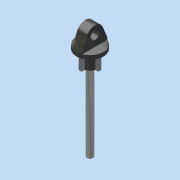
# Autodesk Inventor part: Shock Mount - Top
Saved by Autodesk Inventor 2011 SP1 (Build 150282100, 282)
## iProperties
Created: 2011-09-22
Part Number: Shock Mount - Top
Document SubType Name: Modeling
Designer: dgitz
Density: 1 g/cm^3
Author: dgitz
Autodesk Inventor part; units mm, degrees
ref_plane "YZ Plane" through (0, 0, 0) normal (1, 0, 0) x (0, 1, 0)
ref_plane "XZ Plane" through (0, 0, 0) normal (0, 1, 0) x (-1, 0, 0)
sketch "Sketch2" plane through (0, 0, 0) normal (0, 1, 0) x (-1, 0, 0)
  circle A0 centre (0, 0) radius 1.9812
  dimension "d0" = 3.9624
  constraints: 1 centre point, 1 coincident
  measures "d0" diameter of A0
extrude "Extrusion1" add sketch "Sketch2" along normal blind 50.8
chamfer "Chamfer1" distance 0.7937 angle 45 1 edges at (1.9812, 0, 0)
sketch "Sketch3" plane through (0, 50.8, 0) normal (0, 1, 0) x (1, 0, 0)
  circle A0 centre (0, 0) radius 1.9812 projected
  circle A1 centre (0, 0) radius 4.445
  dimension "d6" = 8.89
  constraints: 1 centre point, 1 coincident
  measures "d6" diameter of A1
extrude "Extrusion2" add sketch "Sketch3" along normal blind 8.89 contours A0 | A1
sketch "Sketch4" plane through (0, 59.69, 0) normal (0, 1, 0) x (1, 0, 0)
  circle A0 centre (0, 0) radius 4.445 projected
  circle A1 centre (0, 0) radius 8.509
  dimension "d9" = 17.018
  constraints: 1 centre point, 1 coincident
  measures "d9" diameter of A1
extrude "Extrusion3" add sketch "Sketch4" along normal blind 2.54 contours A0 | A1
sketch "Sketch5" plane through (0, 0, 0) normal (1, 0, 0) x (0, 1, 0)
  circle A0 centre (68.707, 0) radius 2.667
  arc A1 (70.7539, -5.0629) -> (70.7539, 5.0629) centre (68.707, 0) ccw
  line L0 (59.69, 8.509) -> (62.23, 8.509) projected
  line L1 (62.23, 8.509) -> (62.23, -8.509) projected
  line L2 (59.69, -8.509) -> (62.23, -8.509) projected
  line L3 (62.23, 8.509) -> (62.23, -8.509)
  line L4 (62.23, -8.509) -> (70.7539, -5.0629)
  line L5 (62.23, 8.509) -> (70.7539, 5.0629)
  line L6 (37.7029, 0) -> (42.6845, 0) construction
  line L7 (74.168, 5.5293) -> (74.168, -0.3965) construction
  point P0 (0, 0)
  dimension "d12" = 5.334
  dimension "d13" = 10.922
  dimension "d14" = 11.938
  constraints: 10 end point, 3 tangent, 2 centre point, 2 perpendicular, 2 point on circle, 2 point on line, 1 coincident, 1 vertical
  measures "d12" diameter of A0
  measures "d13" diameter of A1
  measures "d14" distance between parallel lines of L1 L7
extrude "Extrusion4" add sketch "Sketch5" along normal mid plane 6.096
sketch "Sketch6" plane through (0, 62.23, 0) normal (0, 1, 0) x (1, 0, 0)
  arc A0 (3.048, -7.9444) -> (3.048, 7.9444) centre (0, 0) ccw projected
  circle A1 centre (0, 0) radius 8.509
  circle A2 centre (0, 0) radius 9.0384
  point P0 (-3.048, 8.509)
  constraints: 2 concentric, 1 centre point, 1 coincident, 3 other
extrude "Extrusion5" cut sketch "Sketch6" along normal blind 12.7
sketch "Sketch7" plane through (0, 59.69, 0) normal (0, -1, 0) x (1, 0, 0)
  circle A0 centre (0, 0) radius 8.509 projected
  circle A1 centre (0, 0) radius 4.445 projected
  arc A2 (-4.3273, 1.016) -> (-4.3273, -1.016) centre (0, 0) ccw
  circle A3 centre (0, 0) radius 4.445 projected
  arc A4 (-6.2682, 1.016) -> (-6.2682, -1.016) centre (0, 0) ccw
  line L0 (-6.2682, 1.016) -> (-4.3273, 1.016)
  line L1 (-6.2682, -1.016) -> (-4.3273, -1.016)
  arc A5 (-1.016, -4.3273) -> (1.016, -4.3273) centre (0, 0) ccw
  arc A6 (-1.016, -6.2682) -> (1.016, -6.2682) centre (0, 0) ccw
  line L2 (-1.016, -6.2682) -> (-1.016, -4.3273)
  line L3 (1.016, -6.2682) -> (1.016, -4.3273)
  arc A7 (4.3273, -1.016) -> (4.3273, 1.016) centre (0, 0) ccw
  arc A8 (6.2682, -1.016) -> (6.2682, 1.016) centre (0, 0) ccw
  line L4 (6.2682, -1.016) -> (4.3273, -1.016)
  line L5 (6.2682, 1.016) -> (4.3273, 1.016)
  arc A9 (1.016, 4.3273) -> (-1.016, 4.3273) centre (0, 0) ccw
  arc A10 (1.016, 6.2682) -> (-1.016, 6.2682) centre (0, 0) ccw
  line L6 (1.016, 6.2682) -> (1.016, 4.3273)
  line L7 (-1.016, 6.2682) -> (-1.016, 4.3273)
  dimension "d19" = 12.7
  dimension "d20" = 2.032
  dimension "d21" = 1.016
  dimension "d24" = 360
  constraints: 18 point on circle, 16 end point, 8 centre point, 2 coincident, 1 concentric, 1 horizontal, 1 parallel, 41 other
  measures "d19" diameter of A4
  measures "d20" distance between parallel lines of L1 L0
  measures "d21" distance from line of A0.centre L0
extrude "Extrusion6" add sketch "Sketch7" along normal blind 8.89 contours A1 L5 A8 L4 | A1 L7 A10 L6 | L3 A6 L2 A1 | A1 L1 A4 L0
ref_plane "Work Plane1" through (0, 74.168, 0) normal (0, 1, 0) x (-1, 0, 0)
body "Solid1"
